Autodesk Fusion 360 part; units mm, degrees
(part 3 of 3)
sketch "Sketch64" plane through (-835, 0, 0) normal (1, 0, 0) x (0, 1, 0)
  line L0 (-155, 150) -> (-155, 125)
  line L1 (-155, 125) -> (220, 125)
  line L2 (220, 125) -> (220, 150)
  line L3 (220, 150) -> (-155, 150)
  line L4 (220, 200) -> (195, 200)
  line L5 (195, 200) -> (195, 225)
  line L6 (195, 225) -> (220, 225)
  line L7 (220, 225) -> (220, 200)
  line L8 (220, 125) -> (195, 125)
  line L9 (195, 125) -> (195, 150)
  line L10 (195, 150) -> (220, 150)
  line L11 (220, 150) -> (220, 125)
  constraint horizontal L4
  constraint vertical L5
  constraint horizontal L6
  constraint vertical L7
  constraint horizontal L8
  constraint vertical L9
  constraint horizontal L10
  constraint vertical L11
  constraint coincident L3 L9.end
  constraint coincident L1.end L2.start
extrude "Extrude45" add sketch "Sketch64" along normal blind 375 contours L1 L2 L3 L8 L9 L10 L11 | L4 L5 L6 L7 bodies 9 in component "bin case (1)"
sketch "Sketch65" plane through (0, 0, 225) normal (0, 0, 1) x (-1, 0, 0)
  line L0 (485, 180) -> (485, 155)
  line L1 (485, 155) -> (835, 155)
  line L2 (835, 155) -> (835, -195)
  line L3 (835, -195) -> (460, -195)
  line L4 (460, -195) -> (460, -220)
  line L5 (460, -220) -> (860, -220)
  line L6 (860, -220) -> (860, 180)
  line L7 (860, 180) -> (485, 180)
  line L8 (460, -195) -> (485, -195)
  line L9 (485, -195) -> (485, -220)
  line L10 (485, -220) -> (460, -220)
  line L11 (460, -220) -> (460, -195)
  dimension "d438" = 25
  constraint horizontal L8
  constraint vertical L9
  constraint horizontal L10
  constraint vertical L11
  constraint coincident L5 L9.end
  constraint coincident L3.end L4.start
  measures "d438" distance of L9 L11
extrude "Extrude46" add sketch "Sketch65" against normal blind 150 contours L3 L4 L5 L8 L9 L10 L11 bodies 9 in component "bin case (1)"
sketch "Sketch66" plane through (0, -180, 0) normal (0, -1, 0) x (1, 0, 0)
  line L0 (-460, 800) -> (265, 800)
  line L1 (265, 800) -> (265, 25)
  line L2 (265, 25) -> (-460, 25)
  line L3 (-460, 25) -> (-460, 800)
  line L4 (1040, 743.125) -> (1015, 743.125)
  line L5 (1015, 743.125) -> (1015, 25)
  line L6 (1015, 25) -> (290, 25)
  line L7 (290, 25) -> (290, 800)
  line L8 (290, 800) -> (1015, 800)
  line L9 (1015, 800) -> (1015, 825)
  line L10 (1015, 825) -> (965, 825)
  line L11 (965, 825) -> (590, 825)
  line L12 (590, 825) -> (215, 825)
  line L13 (215, 825) -> (-460, 825)
  line L14 (-460, 825) -> (-460, 875)
  line L15 (-460, 875) -> (975, 875)
  line L16 (975, 875) -> (975, 887.5)
  line L17 (975, 887.5) -> (1010, 887.5)
  line L18 (1010, 887.5) -> (1010, 875)
  line L19 (1010, 875) -> (1015, 875)
  line L20 (1015, 875) -> (1015, 865)
  line L21 (1015, 865) -> (1040, 865)
  line L22 (1040, 865) -> (1040, 885)
  line L23 (1040, 885) -> (1015, 885)
  line L24 (1015, 885) -> (1015, 900)
  line L25 (1015, 900) -> (-460, 900)
  line L26 (-460, 900) -> (-485, 900)
  line L27 (-485, 900) -> (-485, 875)
  line L28 (-485, 875) -> (-485, 825)
  line L29 (-485, 825) -> (-486, 825)
  line L30 (-486, 825) -> (-519.6212, 807.8463)
  arc A0 (-519.6212, 807.8463) -> (-535, 775.0001) centre (-534.95, 795) ccw
  line L31 (-535, 775.0001) -> (-535, 775)
  line L32 (-535, 775) -> (-534.9999, 775.0001)
  arc A1 (-534.9999, 775.0001) -> (-518.7278, 783.3022) centre (-534.95, 795) ccw
  line L33 (-518.7278, 783.3022) -> (-486, 800)
  line L34 (-486, 800) -> (-485, 800)
  line L35 (-485, 800) -> (-485, 225)
  line L36 (-485, 225) -> (-860, 225)
  line L37 (-860, 225) -> (-860, 200)
  line L38 (-860, 200) -> (-485, 200)
  line L39 (-485, 200) -> (-485, 150)
  line L40 (-485, 150) -> (-860, 150)
  line L41 (-860, 150) -> (-860, 125)
  line L42 (-860, 125) -> (-485, 125)
  line L43 (-485, 125) -> (-485, 0)
  line L44 (-485, 0) -> (1040, 0)
  line L45 (1040, 0) -> (1040, 743.125)
  line L46 (-485, 190) -> (-460, 190)
  line L47 (-460, 190) -> (-460, 165)
  line L48 (-460, 165) -> (-485, 165)
  line L49 (-485, 165) -> (-485, 190)
  dimension "d441" = 25
  dimension "d442" = 10
  constraint horizontal L46
  constraint vertical L47
  constraint horizontal L48
  constraint vertical L49
  constraint coincident L39 L46.start
  measures "d441" distance of L46.start L48.end
  measures "d442" distance of L38 L46
extrude "Extrude47" add sketch "Sketch66" against normal blind 280 contours L3 L39 L46 L47 L48 L49 bodies 9 in component "bin case (1)"
sketch "Sketch67" plane through (0, 0, 900) normal (0, 0, 1) x (-1, 0, 0)
  line L0 (394.6718, -186.496) -> (414.4306, -172.6608)
  line L1 (414.4306, -172.6608) -> (250, 62.1704)
  line L2 (250, 62.1704) -> (250, 155)
  line L3 (250, 155) -> (485, 155)
  line L4 (485, 155) -> (485, 180)
  line L5 (485, 180) -> (460, 180)
  line L6 (460, 180) -> (-1015, 180)
  line L7 (-1015, 180) -> (-1015, 220)
  line L8 (-1015, 220) -> (-1015, 245)
  line L9 (-1015, 245) -> (-1015, 510)
  line L10 (-1015, 510) -> (-1040, 510)
  line L11 (-1040, 510) -> (-1040, 155)
  line L12 (-1040, 155) -> (160, 155)
  line L13 (160, 155) -> (394.6718, -186.496)
  line L14 (225, 97.8741) -> (185, 155)
  line L15 (185, 155) -> (225, 155)
  line L16 (225, 155) -> (225, 97.8741)
  line L17 (160, 155) -> (419.3003, 155)
  line L18 (419.3003, 155) -> (419.3003, -186.496)
  line L19 (419.3003, -186.496) -> (160, -186.496)
  line L20 (160, -186.496) -> (160, 155)
  constraint horizontal L17
  constraint vertical L18
  constraint horizontal L19
  constraint vertical L20
  constraint coincident L12.end L13.start
extrude "Extrude48" cut sketch "Sketch67" against normal blind 70 contours L0 L1 L2 L13 L14 L16 L17 | L13 L19 L20 | L0 L1 L2 L3 L17 L18 L19 | L14 L15 L16 L17 bodies 9 in component "bin case (1)"
sketch "Sketch68" plane through (0, -155, 0) normal (0, 1, 0) x (-1, 0, 0)
  line L0 (166.0668, 875) -> (460, 875)
  line L1 (460, 875) -> (460, 825)
  line L2 (460, 825) -> (-215, 825)
  line L3 (-215, 825) -> (-590, 825)
  line L4 (-590, 825) -> (-965, 825)
  line L5 (-965, 825) -> (-1015, 825)
  line L6 (-1015, 825) -> (-1015, 875)
  line L7 (-1015, 875) -> (160, 875)
  line L8 (160, 875) -> (160, 831)
  line L9 (160, 831) -> (166.0668, 831)
  line L10 (166.0668, 831) -> (166.0668, 875)
  line L11 (485, 900) -> (-1040, 900)
  line L12 (-1040, 900) -> (-1040, 825)
  line L13 (-1040, 825) -> (-1220, 825)
  line L14 (-1220, 825) -> (-1250.0621, 808.2988)
  arc A0 (-1248.0189, 784.434) -> (-1250.0621, 808.2988) centre (-1265, 795) ccw
  line L15 (-1248.0189, 784.434) -> (-1220, 800)
  line L16 (-1220, 800) -> (-1040, 800)
  line L17 (-1040, 800) -> (-1040, 25)
  line L18 (-1040, 25) -> (-1015, 25)
  line L19 (-1015, 25) -> (-1015, 800)
  line L20 (-1015, 800) -> (-290, 800)
  line L21 (-290, 800) -> (-290, 25)
  line L22 (-290, 25) -> (-265, 25)
  line L23 (-265, 25) -> (-265, 800)
  line L24 (-265, 800) -> (460, 800)
  line L25 (460, 800) -> (460, 190)
  line L26 (460, 190) -> (485, 190)
  line L27 (485, 190) -> (485, 200)
  line L28 (485, 200) -> (835, 200)
  line L29 (835, 200) -> (835, 225)
  line L30 (835, 225) -> (485, 225)
  line L31 (485, 225) -> (485, 800)
  line L32 (485, 800) -> (486, 800)
  line L33 (486, 800) -> (518.7278, 783.3022)
  arc A1 (519.6212, 807.8463) -> (518.7278, 783.3022) centre (534.95, 795) ccw
  line L34 (519.6212, 807.8463) -> (486, 825)
  line L35 (486, 825) -> (485, 825)
  line L36 (485, 825) -> (485, 875)
  line L37 (485, 875) -> (485, 900)
  line L38 (160, 875) -> (166.0668, 875)
  line L39 (166.0668, 875) -> (166.0668, 831)
  line L40 (166.0668, 831) -> (160, 831)
  line L41 (160, 831) -> (160, 875)
  constraint horizontal L38
  constraint vertical L39
  constraint horizontal L40
  constraint vertical L41
  constraint coincident L9.end L10.start
  constraint coincident L7.end L8.start
extrude "Extrude49" cut sketch "Sketch68" against normal blind 10 contours L8 L9 L10 L38 L39 L40 L41 bodies 9 in component "bin case (1)"
sketch "Sketch69" plane through (0, 0, 825) normal (0, 0, 1) x (-1, 0, 0)
  arc A0 (-215, 155) -> (-215, 180) centre (-215, 167.5) ccw
  line L0 (-215, 155) -> (460, 155)
  line L1 (460, 155) -> (460, 180)
  line L2 (460, 180) -> (-215, 180)
  circle A1 centre (167.3818, 167.5) radius 12.5
  constraint tangent L2 A1
extrude "Extrude50" add sketch "Sketch69" along normal blind 10 contours A1 bodies 9 in component "bin case (1)"
sketch "Sketch70" plane through (0, 0, 835) normal (0, 0, 1) x (-1, 0, 0)
  circle A0 centre (167.3818, 167.5) radius 12.5
  circle A1 centre (167.3818, 167.5) radius 17.5
  dimension "d451" = 35
  constraint concentric A0 A1
  measures "d451" diameter of A1
extrude "Extrude1'''''''''''''" add sketch "Sketch70" along normal blind 40 separate body contours A0 | A1 makes body 35 in component "redPaddle"
sketch "Sketch71" plane through (0, 0, 875) normal (0, 0, 1) x (-1, 0, 0)
  circle A0 centre (167.3818, 167.5) radius 17.5
sketch "Sketch72" plane through (0, 0, 875) normal (0, 0, 1) x (-1, 0, 0)
  circle A0 centre (167.3818, 167.5) radius 17.5
  circle A1 centre (167.3818, 167.5) radius 10
  line L0 (167.3818, 157.5) -> (167.3818, 177.5)
  line L1 (167.3818, 177.5) -> (447.3818, 177.5)
  line L2 (447.3818, 177.5) -> (447.3818, 157.5)
  line L3 (447.3818, 157.5) -> (167.3818, 157.5)
  dimension "d454" = 20
  dimension "d455" = 280
  constraint concentric A0 A1
  constraint perpendicular L0 L1
  constraint parallel L0 L2
  constraint parallel L1 L3
  constraint coincident A1 L0.end
  constraint vertical L0
  constraint coincident A1 L0.start
  measures "d454" diameter of A1
  measures "d455" distance of L0.start L2.end
extrude "Extrude8'" add sketch "Sketch72" against normal blind 40 separate body contours A0 L1 L2 L3 makes body 36
copy_body "CutPasteBodies1'''" bodies 36 removing the originals makes body 37 in component "redPaddle"
sketch "Sketch73" plane through (1275, 0, 0) normal (1, 0, 0) x (0, 1, 0)
  line L0 (-220.0236, 874.9783) -> (-209.7761, 869.9181)
  arc A0 (-209.7761, 869.9181) -> (-195, 887.5) centre (-195, 872.5) ccw
  line L1 (-195, 887.5) -> (-195, 887.6217)
  line L2 (-195, 887.6217) -> (-220.0236, 899.9783)
  line L3 (-220.0236, 899.9783) -> (-510.0236, 899.9783)
  line L4 (-510.0236, 899.9783) -> (-538.2278, 885.8842)
  arc A1 (-538.2278, 885.8842) -> (-533.0041, 863.4946) centre (-545, 872.5) ccw
  line L5 (-533.0041, 863.4946) -> (-510.0236, 874.9783)
  line L6 (-510.0236, 874.9783) -> (-245.0236, 874.9783)
  line L7 (-245.0236, 874.9783) -> (-245.0236, 799.9783)
  line L8 (-245.0236, 799.9783) -> (-220.0236, 799.9783)
  line L9 (-220.0236, 799.9783) -> (-220.0236, 874.9783)
  circle A2 centre (-500.0236, 894.9783) radius 3
  dimension "d464" = 6
  dimension "d465" = 5
  dimension "d466" = 10
  measures "d464" diameter of A2
  measures "d465" distance of L3 A2.centre
  measures "d466" horizontal distance of L3.end A2.centre
extrude "Extrude1''''''''''''''" add sketch "Sketch73" against normal blind 260 separate body contours A2 makes body 38 in component "printerCore"
ref_plane "WorkPlane3" through (1145, -500.0236, 894.9783) normal (1, 0, 0) x (0, 1, 0)
sketch "Sketch74" plane through (1145, 0, 0) normal (1, 0, 0) x (0, 1, 0)
  circle A0 centre (-500, 895) radius 6
extrude "Extrude9'" add sketch "Sketch74" along normal mid plane 20 separate body makes body 39
copy_body "CutPasteBodies1''''" bodies 39 removing the originals makes body 40 in component "printerCore"
ref_plane "WorkPlane4" through (1185, -500.0236, 894.9783) normal (1, 0, 0) x (0, 1, 0)
mirror "Mirror1" about plane through (1185, -500.0236, 894.9783) normal (1, 0, 0) of bodies 40 makes body 41 in component "printerCore"
ref_plane "WorkPlane5" through (1105, -500.0236, 894.9783) normal (1, 0, 0) x (0, 1, 0)
mirror "Mirror2" about plane through (1105, -500.0236, 894.9783) normal (1, 0, 0) of bodies 40 makes body 42 in component "printerCore"
pattern_linear "00000000-0000-0000-0000-000000000000" [suppressed]
component "belt sensor" placed x (1, 0, 0) y (0, 1, 0) z (0, 0, 1) at (-355, 75, 87.5)
component "belt" placed x (1, 0, 0) y (0, 1, 0) z (0, 0, 1) at (-374.9325, 80, 10)
component "power" placed x (1, 0, 0) y (0, 1, 0) z (0, 0, 1) at (-459.9325, 75, 25)
component "vibrator" placed x (1, 0, 0) y (0, 1, 0) z (0, 0, 1) at (0, 0, 0)
component "bin case" placed x (1, 0, 0) y (0, 1, 0) z (0, 0, 1) at (0, 0, 0)
component "bin case (1)" placed x (1, 0, 0) y (0, 1, 0) z (0, 0, 1) at (0, 0, 0)
component "motor belt" placed x (1, 0, 0) y (0, 1, 0) z (0, 0, 1) at (0.0675, 0, 0)
component "case lock" placed x (1, 0, 0) y (0, -1, 0) z (0, 0, -1) at (0, 925, 1625)
component "case lock" placed x (1, 0, 0) y (0, -1, 0) z (0, 0, -1) at (375, 925, 1625)
component "case lock" placed x (1, 0, 0) y (0, -1, 0) z (0, 0, -1) at (750, 925, 1625)
component "case lock" placed x (1, 0, 0) y (0, -1, 0) z (0, 0, -1) at (1125, 925, 1625)
component "mortor b2" placed x (1, 0, 0) y (0, 1, 0) z (0, 0, 1) at (0, 0, 0)
component "cam" placed x (1, 0, 0) y (0, 1, 0) z (0, 0, 1) at (0, 25, 0)
component "paddle1" placed x (1, 0, 0) y (0, 1, 0) z (0, 0, 1) at (0, 0, 0)
component "paddle1" placed x (1, 0, 0) y (0, 1, 0) z (0, 0, 1) at (375, 0, 0)
component "paddle1" placed x (1, 0, 0) y (0, 1, 0) z (0, 0, 1) at (750, 0, 0)
component "bin" placed x (1, 0, 0) y (0, 1, 0) z (0, 0, 1) at (0, 0, 0)
component "bin (1)" placed x (1, 0, 0) y (0, 1, 0) z (0, 0, 1) at (-375, 0, 0)
component "bin (2)" placed x (1, 0, 0) y (0, 1, 0) z (0, 0, 1) at (-750, 0, 0)
component "bin (3)" placed x (1, 0, 0) y (0, 1, 0) z (0, 0, 1) at (-1125, 0, 0)
component "limit" placed x (1, 0, 0) y (0, 1, 0) z (0, 0, 1) at (0, 0, 0)
component "bin (4)" placed x (1, 0, 0) y (0, 1, 0) z (0, 0, 1) at (-1508.3056, -280.1892, -21.425)
component "redPaddle" placed x (1, 0, 0) y (0, 1, 0) z (0, 0, 1) at (0, 0, 0)
component "printerCore" placed x (1, 0, 0) y (0, 1, 0) z (0, 0, 1) at (0, 0, 0)
component "printerCore" placed x (1, 0, 0) y (0, 1, 0) z (0, 0, 1) at (0, 90, 0)
component "printerCore" placed x (1, 0, 0) y (0, 1, 0) z (0, 0, 1) at (0, 180, 0)
component "printerCore" placed x (1, 0, 0) y (0, 1, 0) z (0, 0, 1) at (0, 270, 0)
